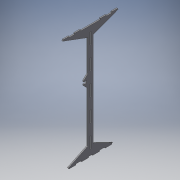
# Autodesk Inventor part: TrayPanelF
Saved by Autodesk Inventor 2017 (Build 210142000, 142)
## iProperties
Created: 2019-06-22
Part Number: TrayPanelF
Material: Generic
Document SubType Name: Modeling
Designer: DDeGo
Density: 1 g/cm^3
Appearance: Default
Author: DDeGo
Autodesk Inventor part; units mm, degrees
ref_plane "YZ Plane" through (0, 0, 0) normal (1, 0, 0) x (0, 1, 0)
ref_plane "XZ Plane" through (0, 0, 0) normal (0, 1, 0) x (-1, 0, 0)
ref_plane "XY Plane" through (0, 0, 0) normal (0, 0, 1) x (1, 0, 0)
sketch "Sketch1" plane through (0, 0, 0) normal (1, 0, 0) x (0, 1, 0)
  line L0 (0, 0) -> (14, 0) construction
  line L1 (14, 0) -> (14, 250)
  line L2 (14, 250) -> (0, 250) construction
  line L3 (0, 250) -> (0, 0)
  line L4 (-50, -25) -> (64, -25)
  line L5 (79, 275) -> (-65, 275)
  line L6 (8.375, 200) -> (5.625, 200)
  line L7 (5.625, 200) -> (5.625, 170)
  line L8 (5.625, 170) -> (8.375, 170)
  line L9 (8.375, 170) -> (8.375, 200)
  line L10 (8.375, 140) -> (5.625, 140)
  line L11 (5.625, 140) -> (5.625, 110)
  line L12 (5.625, 110) -> (8.375, 110)
  line L13 (8.375, 110) -> (8.375, 140)
  line L14 (8.375, 80) -> (5.625, 80)
  line L15 (5.625, 80) -> (5.625, 50)
  line L16 (5.625, 50) -> (8.375, 50)
  line L17 (8.375, 50) -> (8.375, 80)
  line L18 (8.375, 20) -> (5.625, 20)
  line L19 (5.625, 20) -> (5.625, -10)
  line L20 (5.625, -10) -> (8.375, -10)
  line L21 (8.375, -10) -> (8.375, 20)
  line L22 (8.375, 230) -> (5.625, 230)
  line L23 (5.625, 230) -> (5.625, 260)
  line L24 (5.625, 260) -> (8.375, 260)
  line L25 (8.375, 260) -> (8.375, 230)
  line L26 (-65, 275) -> (-49.85, 275)
  line L27 (-49.85, 275) -> (-49.85, 277.75)
  line L28 (-49.85, 277.75) -> (-65, 277.75)
  line L29 (-65, 277.75) -> (-65, 275)
  line L30 (79, 275) -> (63.85, 275)
  line L31 (63.85, 275) -> (63.85, 277.75)
  line L32 (63.85, 277.75) -> (79, 277.75)
  line L33 (79, 277.75) -> (79, 275)
  line L34 (-34.85, 275) -> (-19.7, 275)
  line L35 (-19.7, 275) -> (-19.7, 277.75)
  line L36 (-19.7, 277.75) -> (-34.85, 277.75)
  line L37 (-34.85, 277.75) -> (-34.85, 275)
  line L38 (33.7, 275) -> (48.85, 275)
  line L39 (48.85, 275) -> (48.85, 277.75)
  line L40 (48.85, 277.75) -> (33.7, 277.75)
  line L41 (33.7, 277.75) -> (33.7, 275)
  line L42 (-50, -25) -> (-31.85, -25)
  line L43 (-31.85, -25) -> (-31.85, -27.75)
  line L44 (-31.85, -27.75) -> (-50, -27.75)
  line L45 (-50, -27.75) -> (-50, -25)
  line L46 (-16.85, -25) -> (1.3, -25)
  line L47 (1.3, -25) -> (1.3, -27.75)
  line L48 (1.3, -27.75) -> (-16.85, -27.75)
  line L49 (-16.85, -27.75) -> (-16.85, -25)
  line L50 (12.7, -25) -> (30.85, -25)
  line L51 (30.85, -25) -> (30.85, -27.75)
  line L52 (30.85, -27.75) -> (12.7, -27.75)
  line L53 (12.7, -27.75) -> (12.7, -25)
  line L54 (64, -25) -> (45.85, -25)
  line L55 (45.85, -25) -> (45.85, -27.75)
  line L56 (45.85, -27.75) -> (64, -27.75)
  line L57 (64, -27.75) -> (64, -25)
  line L58 (0, 250) -> (-67, 275)
  line L59 (-67, 275) -> (-65, 275)
  line L60 (79, 275) -> (81, 275)
  line L61 (81, 275) -> (14, 250)
  line L62 (-50, -25) -> (-52, -25)
  line L63 (-52, -25) -> (0, 0)
  line L64 (64, -25) -> (66, -25)
  line L65 (66, -25) -> (14, 0)
  point P0 (7, 170)
  dimension "d3" = 30
  dimension "d4" = 60
  dimension "d5" = 60
  dimension "d6" = 60
  dimension "d7" = 7
  dimension "d8" = 7
  dimension "d9" = 2.75
  dimension "d10" = 15
  dimension "d11" = 50
  dimension "d12" = 50
  dimension "d13" = 25
  dimension "d14" = 25
  dimension "d15" = 65
  dimension "d16" = 300
  dimension "d17" = 65
  dimension "d18" = 60
  dimension "d19" = 2.75
  dimension "d21" = 15.15
  dimension "d22" = 15
  dimension "d24" = 15
  dimension "d27" = 2.75
  dimension "d28" = 18.15
  dimension "d29" = 15
  dimension "d30" = 15
  dimension "d31" = 11.4
  dimension "d32" = 30.15
  dimension "d34" = 68.55
  dimension "d35" = 30.15
  dimension "d44" = 2
  dimension "d45" = 2
  dimension "d46" = 2
  dimension "d47" = 2
  constraints: 132 end point, 29 parallel, 18 horizontal, 15 point on line, 14 collinear, 14 perpendicular, 1 midpoint
  measures "d3" distance of L8.end L6.start
  measures "d4" distance between parallel lines of L10 L6
  measures "d5" distance of L14.start L10.start
  measures "d6" distance between parallel lines of L14 L18
  measures "d7" distance from line of L3 point (7, 170)
  measures "d8" distance from line of L1 point (7, 170)
  measures "d9" distance of L7.end L8.end
  measures "d10" distance between parallel lines of L4 L20
  measures "d11" distance from line of L4.start L3
  measures "d12" distance from line of L4.end L1
  measures "d13" distance between parallel lines of L4 L0
  measures "d14" distance between parallel lines of L5 L2
  measures "d15" distance from line of L1 L5.start
  measures "d16" distance between parallel lines of L4 L5
  measures "d17" distance from line of L3 L5.end
  measures "d18" distance of L24.end L6.start
  measures "d19" distance of L28.end L5.end
  measures "d21" distance of L31.end L32.end
  measures "d22" distance between parallel lines of L39 L31
  measures "d24" distance between parallel lines of L27 L37
  measures "d27" distance of L56.end L4.end
  measures "d28" distance of L55.end L56.end
  measures "d29" distance of L51.end L55.end
  measures "d30" distance of L48.end L43.end
  measures "d31" distance between parallel lines of L47 L53
  measures "d32" distance of L39.end L32.end
  measures "d34" distance from line of L35 L39.end
  measures "d35" distance of L35.end L27.end
  measures "d44" distance of L58.end L5.end
  measures "d45" distance of L5.start L60.end
  measures "d46" distance of L4.end L64.end
  measures "d47" distance of L4.start L62.end
extrude "Extrusion1" add sketch "Sketch1" along normal blind 2.75
sketch "Sketch2" plane through (0, 0, 0) normal (-1, 0, 0) x (0, 0, 1)
  line L0 (250, 0) -> (0, 0) projected
  line L1 (166.85, 0) -> (155.85, -11)
  line L2 (155.85, -11) -> (152.85, -11)
  line L3 (152.85, -11) -> (152.85, -3)
  line L4 (152.85, -3) -> (147.25, -3)
  line L5 (147.25, -3) -> (147.25, -11)
  line L6 (147.25, -11) -> (144.25, -11)
  line L7 (144.25, -11) -> (133.25, 0)
  line L8 (-27.75, -50) -> (-27.75, -31.85) projected
  dimension "d36" = 8
  dimension "d38" = 5.6
  dimension "d39" = 11
  dimension "d40" = 45
  dimension "d41" = 3
  dimension "d48" = 175
  constraints: 14 end point, 4 point on line, 3 perpendicular, 2 equal length, 1 parallel
  measures "d36" distance between parallel lines of L6 L4
  measures "d38" distance of L3.end L4.end
  measures "d39" distance between parallel lines of L0 L6
  measures "d40" angle of L0 L7
  measures "d41" distance of L5.end L6.end
  measures "d48" distance between parallel lines of L8 L5
extrude "Extrusion2" add sketch "Sketch2" against normal up to surface (2.75 mm away)
equation "\"d5\" = d4"
equation "\"d6\" = d4"
equation "\"d18\" = d4"
equation "\"d30\" = d29"
body "Solid1"
